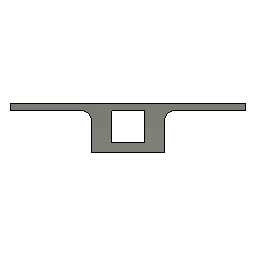
battery_holder (Autodesk Fusion 360 design; units mm, degrees)
Autodesk Fusion 360 part; units mm, degrees
sketch "Sketch1" plane through (0, 0, 0) normal (0, 1, 0) x (1, 0, 0)
  line L0 (-50, 5) -> (15, 5)
  line L1 (15, 5) -> (15, -40)
  line L2 (15, -40) -> (-50, -40)
  line L3 (-50, -40) -> (-50, 5)
  dimension "d1" = 65
  dimension "d2" = 45
  constraint horizontal L0
  constraint vertical L1
  constraint horizontal L2
  constraint vertical L3
  measures "d1" distance of L0.start L0.end
  measures "d2" distance of L0.start L2.end
extrude "Extrude1" add sketch "Sketch1" along normal blind 2
sketch "Sketch2" plane through (0, 2, 0) normal (0, 1, 0) x (-1, 0, 0)
  line L0 (50, 40) -> (-15, 40)
  line L1 (-15, 40) -> (-15, -5)
  line L2 (-15, -5) -> (50, -5)
  line L3 (50, -5) -> (50, 40)
  line L4 (50, 17.5) -> (-15, 17.5)
  line L5 (50, 14.5) -> (-15, 14.5)
  line L6 (-15, 20.5) -> (50, 20.5)
  line L7 (50, 12.5) -> (-15, 12.5)
  line L8 (-15, 22.5) -> (50, 22.5)
  line L9 (50, 17.5) -> (40, 17.5)
  line L10 (40, 17.5) -> (40, 12.5)
  line L11 (40, 17.5) -> (40, 22.5)
  line L12 (-15, 17.5) -> (-5, 17.5)
  line L13 (-5, 17.5) -> (-5, 12.5)
  line L14 (-5, 17.5) -> (-5, 22.5)
  dimension "d5" = 3
  dimension "d6" = 6
  dimension "d7" = -2
  dimension "d8" = -2
  dimension "d9" = 10
  dimension "d15" = 10
  constraint midpoint L1 L4.end
  constraint horizontal L5
  constraint horizontal L6
  constraint perpendicular L3 L9
  constraint coincident L7 L10.end
  constraint perpendicular L7 L10
  constraint coincident L8 L11.end
  constraint perpendicular L8 L11
  constraint perpendicular L1 L12
  constraint coincident L7 L13.end
  constraint perpendicular L7 L13
  constraint coincident L8 L14.end
  constraint perpendicular L8 L14
  measures "d5" distance of L4.start L5.start
  measures "d6" distance of L5.start L6.end
  measures "d9" distance of L4.start L9.end
  measures "d15" distance of L4.end L12.end
extrude "Extrude2" add sketch "Sketch2" along normal blind 7 contours L3 L6 L8 L11 | L3 L5 L7 L10
sketch "Sketch3" plane through (0, 0, 14.5) normal (0, 0, 1) x (1, 0, 0)
  line L0 (-50, 2) -> (-40, 2)
  line L1 (-40, 2) -> (-40, 9)
  line L2 (-40, 9) -> (-50, 9)
  line L3 (-50, 9) -> (-50, 2)
  line L4 (-40, 8) -> (-50, 8)
  dimension "d12" = -1
extrude "Extrude4" add sketch "Sketch2" along normal blind 7 contours L1 L6 L8 L14 | L1 L5 L7 L13
sketch "Sketch4" plane through (0, 0, 14.5) normal (0, 0, 1) x (1, 0, 0)
  line L0 (5, 2) -> (15, 2)
  line L1 (15, 2) -> (15, 9)
  line L2 (15, 9) -> (5, 9)
  line L3 (5, 9) -> (5, 2)
  line L4 (15, 8) -> (5, 8)
  dimension "d18" = -1
extrude "Extrude5" add sketch "Sketch4" along normal blind 6 contours L1 L2 L3 L4
extrude "Extrude6" add 1 faces at (8.3333, 9, 19.1667) along direction (0, 1, 0) blind 1
extrude "Extrude7" add sketch "Sketch3" along normal blind 1 contours L1 L2 L3 L4
extrude "Extrude8" add 1 faces at (-46.6667, 8.6667, 15.5) along direction (0, 0, 1) blind 5
extrude "Extrude9" add 1 faces at (-43.3333, 9, 15.8333) along direction (0, 1, 0) blind 1
extrude "Extrude10" cut 1 faces at (-28.3333, 0, 10) along direction (0, 1, 0) blind 0.5
sketch "Sketch5" plane through (0, 0, 22.5) normal (0, 0, 1) x (1, 0, 0)
  line L0 (-50, 2) -> (-40, 2)
  line L1 (-40, 2) -> (-40, 10)
  line L2 (-40, 10) -> (-50, 10)
  line L3 (-50, 10) -> (-50, 2)
  line L4 (-50, 2) -> (-50, 2.3478)
  circle A0 centre (-45, 5) radius 1
  dimension "d31" = 2
  constraint coincident L0.start L3.end
  constraint coincident L3 L4.end
  measures "d31" diameter of A0
hole "Hole1" at (-45, 5, 22.5) direction (0, 0, -1) diameter 2 depth 2 tip angle 180
sketch "Sketch6" plane through (0, 0, 12.5) normal (0, 0, -1) x (-1, 0, 0)
  line L0 (40, 2) -> (50, 2)
  line L1 (50, 2) -> (50, 10)
  line L2 (50, 10) -> (40, 10)
  line L3 (40, 10) -> (40, 2)
  line L4 (40, 2) -> (45, 2)
  line L5 (45, 2) -> (45, 5)
  circle A0 centre (45, 5) radius 1
  dimension "d35" = 3
  dimension "d36" = 2
  constraint coincident L0.start L3.end
  constraint midpoint L0 L4.end
  constraint perpendicular L4 L5
  constraint coincident L5.end A0.centre
  measures "d35" distance of L4.end L5.end
  measures "d36" diameter of A0
hole "Hole2" at (-45, 5, 12.5) direction (0, 0, 1) diameter 2 depth 2 tip angle 180
sketch "Sketch7" plane through (0, 0, 12.5) normal (0, 0, -1) x (-1, 0, 0)
  line L0 (-15, 2) -> (-5, 2)
  line L1 (-5, 2) -> (-5, 10)
  line L2 (-5, 10) -> (-15, 10)
  line L3 (-15, 10) -> (-15, 2)
  line L4 (-15, 2) -> (-10, 2)
  line L5 (-10, 2) -> (-10, 5)
  circle A0 centre (-10, 5) radius 1
  dimension "d40" = 3
  dimension "d41" = 2
  constraint coincident L0.start L3.end
  constraint midpoint L0 L4.end
  constraint perpendicular L4 L5
  constraint coincident L5.end A0.centre
  measures "d40" distance of L4.end L5.end
  measures "d41" diameter of A0
hole "Hole3" at (10, 5, 12.5) direction (0, 0, 1) diameter 2 depth 2 tip angle 180
sketch "Sketch8" plane through (0, 2, 0) normal (0, 1, 0) x (-1, 0, 0)
sketch "Sketch9" plane through (0, 0, 22.5) normal (0, 0, 1) x (1, 0, 0)
  line L0 (5, 2) -> (15, 2)
  line L1 (15, 2) -> (15, 10)
  line L2 (15, 10) -> (5, 10)
  line L3 (5, 10) -> (5, 2)
  line L4 (5, 2) -> (10, 2)
  line L5 (10, 2) -> (10, 5)
  circle A0 centre (10, 5) radius 1
  dimension "d45" = 3
  dimension "d46" = 2
  constraint coincident L0.start L3.end
  constraint midpoint L0 L4.end
  constraint perpendicular L4 L5
  constraint coincident L5.end A0.centre
  measures "d45" distance of L4.end L5.end
  measures "d46" diameter of A0
hole "Hole4" at (10, 5, 22.5) direction (0, 0, -1) diameter 2 depth 2 tip angle 180
fillet "Fillet1" radius 1.5 4 edges at (-45, 2, 12.5) (-45, 2, 22.5) (10, 2, 22.5) (10, 2, 12.5)
delete_face "DeleteFace1" 4 faces at (-43.3333, 2.1667, 23.3127) (-46.6667, 2.5728, 12.1791) (8.3333, 3.4286, 12.4983) (11.6667, 3.4286, 22.5017)
move_face "OffsetFaces1" offset -0.1 3 faces at (-10, 2, 34.1667) (11.6667, 8, 16.5) (-46.6667, 8, 18.5)
move_face "OffsetFaces2" offset -0.1 4 faces at (-41.3343, 4.9751, 20.5) (-41.3343, 4.9751, 14.5) (6.3343, 5.0249, 14.5) (13.6657, 5.0249, 20.5)
fillet "Fillet2" radius 2 4 edges at (-45, 1.9, 12.5) (10, 1.9, 12.5) (10, 1.9, 22.5) (-45, 1.9, 22.5)
move_body "Move1" bodies 1 to x (1, 0, 0) y (0, 1, 0) z (0, 0, 1) at (17.5, -1.9, -17.5)
move_body "Move2" bodies 1 to x (1, 0, 0) y (0, -1, 0) z (0, 0, -1) at (0, 0, 0)
move_body "Move3" bodies 1 to x (1, 0, 0) y (0, 1, 0) z (0, 0, 1) at (0, 3, 0)
move_body "Move4" bodies 1 to x (1, 0, 0) y (0, 0, 1) z (0, -1, 0) at (0, 0, 0)
delete_face "DeleteFace2" 4 faces at (25.8333, -5.0023, 1.0952) (29.1667, 5.0023, 1.0952) (-29.1667, 5.2679, 2) (-25.8333, -6.9048, 2.9977)
move_face "OffsetFaces3" offset 2 4 faces at (-27.5, -5, -3.7667) (27.5, -5, -3.7667) (27.5, 5, -3.7667) (-27.5, 5, -3.7667)
fillet "Fillet3" radius 2 4 edges at (27.5, -7, 3) (-27.5, -7, 3) (-27.5, 7, 3) (27.5, 7, 3)
extrude "Extrude3" [suppressed]
equation "d52 = ( -0.2 / 2 ) * 1 mm"
equation "d53 = ( -0.2 / 2 ) * 1 mm"
